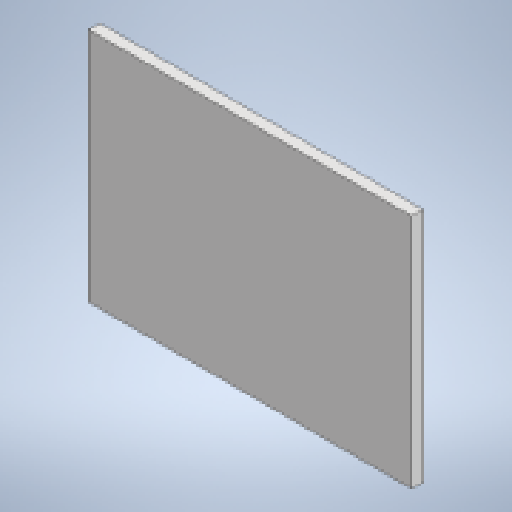
# Autodesk Inventor part: Lateral izquierdo
Saved by Autodesk Inventor 2024 (Build 280153000, 153)
## iProperties
Created: 2025-03-02
Part Number: Lateral izquierdo
Material: Genérico
Document SubType Name: Modeling
Designer: sergi
Density: 1 g/cm^3
Appearance: Valor por defecto
Author: sergi
Autodesk Inventor part; units mm, degrees
ref_plane "YZ Plane" through (0, 0, 0) normal (1, 0, 0) x (0, 1, 0)
ref_plane "XZ Plane" through (0, 0, 0) normal (0, 1, 0) x (-1, 0, 0)
ref_plane "XY Plane" through (0, 0, 0) normal (0, 0, 1) x (1, 0, 0)
sketch "Boceto1" plane through (0, 0, 0) normal (0, 0, 1) x (1, 0, 0)
  line L0 (30, -83.65) -> (30, 0) projected
  line L1 (0, 0) -> (30, 0) projected
  line L2 (0, 0) -> (0, -83.65) projected
  line L3 (0, -83.65) -> (30, -83.65) projected
  line L4 (-13.92, -24.65) -> (-9.92, -24.65) projected
  line L5 (30, -83.65) -> (-55, -83.65)
  line L6 (-55, -83.65) -> (-55, -24.65)
  line L7 (-55, -24.65) -> (30, -24.65)
  line L8 (30, -24.65) -> (30, -83.65)
  line L9 (-55, -24.65) -> (-55, -21.65)
  line L10 (-55, -21.65) -> (30, -21.65)
  line L11 (0, -83.65) -> (10, -83.65)
  line L12 (10, -83.65) -> (10, -21.65)
  circle A0 centre (5, -78.65) radius 2.1 projected
  circle A1 centre (5, -26.65) radius 2.1 projected
  dimension "d0" = 85
  dimension "d1" = 59
  dimension "d2" = 3
  dimension "d5" = 10
  constraints: 16 end point, 3 perpendicular, 3 point on line, 2 parallel, 1 horizontal, 1 vertical
  measures "d0" distance of L6.end L7.end
  measures "d1" distance of L5.end L6.end
  measures "d2" distance of L6.end L9.end
  measures "d5" distance of L2.end L11.end
extrude "Extrusión1" add sketch "Boceto1" along normal blind 6 contours L3 L2 L7 A1 L12 | L7 A1 L2 L10 L12 | L5 L6 L7 L4 L2 | A1 L7 | L7 A1 | L7 L4 L9 L10 L2 | A0
sketch "Boceto2" plane through (0, 0, 6) normal (0, 0, 1) x (1, 0, 0)
  line L0 (10, -83.65) -> (10, -21.65) projected
  line L1 (-55, -83.65) -> (10, -83.65) projected
  line L2 (10, -21.65) -> (-55, -21.65) projected
  point P0 (0, 0)
  point P1 (5, -78.65)
  point P2 (5, -26.65)
  dimension "d6" = 5
  dimension "d7" = 5
  dimension "d8" = 5
  dimension "d9" = 5
  measures "d6" distance from line of L0 point (5, -78.65)
  measures "d7" distance from line of L1 point (5, -78.65)
  measures "d8" distance from line of L2 point (5, -26.65)
  measures "d9" distance from line of L0 point (5, -26.65)
hole "Agujero1" at (5, -78.65, 6) at (5, -26.65, 6) direction (0, 0, -1) diameter 3.2 end through all
sketch "Boceto3" plane through (0, 0, 0) normal (0, 0, -1) x (-1, 0, 0)
  circle A0 centre (-5, -78.65) radius 2.1
  circle A1 centre (-5, -26.65) radius 2.1
  line L0 (-12, 0) -> (-12, -7.15)
  line L1 (-12, -7.15) -> (-30, -7.15)
  line L2 (-30, -7.15) -> (-30, -83.65)
  line L3 (0, -83.65) -> (-30, -83.65)
  line L4 (0, -83.65) -> (0, 0)
  line L5 (0, 0) -> (-12, 0)
  line L6 (20.12, -21.65) -> (-10, -21.65)
  line L7 (-10, -21.65) -> (-10, -83.65)
  circle A2 centre (-5, -26.65) radius 1.6
  circle A3 centre (-5, -78.65) radius 1.6
  circle A4 centre (-5, -26.65) radius 1.6 projected
  circle A5 centre (-5, -78.65) radius 1.6 projected
  line L8 (55, -21.65) -> (55, -83.65) projected
  line L9 (-10, -21.65) -> (55, -21.65) projected
  line L10 (-10, -83.65) -> (-10, -21.65) projected
  line L11 (55, -83.65) -> (-10, -83.65) projected
  line L12 (-10, -83.65) -> (20.12, -83.65)
  line L13 (20.12, -83.65) -> (20.12, -21.65)
  point P0 (0, -21.65)
  constraints: 20 end point, 4 centre point
extrude "Extrusión2" cut sketch "Boceto3" against normal blind 3 contours A0 | A1 | L5 L4 L6 L7 L3 L2 L1 L0 | L6 L13 L11 L4 | L4 L3 L7 L6 | L9 L8 L11 L13 | A2 | A3
sketch "Boceto4" plane through (-55, -21.65, 6) normal (0, 1, 0) x (1, 0, 0)
  line L0 (65, 3) -> (0, 3) projected
  line L1 (0, 3) -> (0, 0) projected
  line L2 (65, 0) -> (0, 0) projected
  line L3 (65, 3) -> (65, 0) projected
  line L4 (0, 0) -> (65, 0)
  line L5 (65, 0) -> (65, 6)
  line L6 (65, 6) -> (0, 6)
  line L7 (0, 6) -> (0, 0)
  point P0 (55, 6)
  constraints: 8 end point, 2 parallel, 1 horizontal, 1 perpendicular
extrude "Extrusión3" add sketch "Boceto4" along normal blind 5
sketch "Boceto5" plane through (-55, -83.65, 3) normal (-1, 0, 0) x (0, 0, 1)
  line L0 (-69, 62) -> (-69, 59)
  line L1 (-3, 59) -> (-69, 59)
  line L2 (-3, 59) -> (-3, 62)
  line L3 (-3, 62) -> (-69, 62)
  line L4 (0, 62) -> (0, 0) projected
  line L5 (0, 0) -> (3, 0) projected
  line L6 (3, 0) -> (3, 67) projected
  line L7 (-3, 67) -> (3, 67) projected
  line L8 (-3, 62) -> (-3, 67) projected
  line L9 (-3, 62) -> (0, 62) projected
  line L10 (-3, 59) -> (3, 59)
  line L11 (3, 59) -> (3, 62)
  line L12 (3, 62) -> (-3, 62)
  line L13 (-3, 62) -> (-3, 59)
  point P0 (-3, 83.65)
  point P1 (0, 59)
  constraints: 16 end point, 2 parallel, 1 horizontal, 1 perpendicular, 1 point on line
extrude "Extrusión4" cut sketch "Boceto5" against normal blind 33.88 contours L12 L6 L10 L4
sketch "Boceto6" plane through (-55, -16.65, 6) normal (0, 1, 0) x (1, 0, 0)
  line L0 (0, 6) -> (0, 0) projected
  line L1 (0, 0) -> (65, 0) projected
  line L2 (65, 0) -> (65, 6) projected
  line L3 (65, 6) -> (0, 6) projected
  line L4 (0, 0) -> (0, 3)
  line L5 (0, 3) -> (3, 3)
  circle A0 centre (3, 3) radius 2.1
  line L6 (33.88, 3) -> (33.88, 0) projected
  line L7 (33.88, 3) -> (30.88, 3)
  circle A1 centre (30.88, 3) radius 2.1
  dimension "d34" = 3
  dimension "d35" = 4.2
  dimension "d36" = 4.2
  constraints: 6 end point, 2 centre point, 2 coincident, 1 horizontal, 1 midpoint, 1 perpendicular
  measures "d34" distance of L0.end L4.end
  measures "d35" diameter of A0
  measures "d36" diameter of A1
hole "Agujero2" at (-52, -16.65, 3) at (-24.12, -16.65, 3) direction (0, -1, 0) diameter 4.2 depth 5
